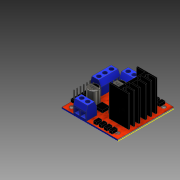
# Autodesk Inventor part: cau h l298
Saved by Autodesk Inventor 2016 (Build 200138000, 138)
## iProperties
Created: 2017-05-27
Part Number: cau h l298
Material: Generic
Document SubType Name: Modeling
Designer: USER
Density: 1 g/cm^3
Appearance: Default
Author: USER
Autodesk Inventor part; units mm, degrees
(part 1 of 2)
ref_plane "YZ Plane" through (0, 0, 0) normal (1, 0, 0) x (0, 1, 0)
sketch "Sketch1" plane through (0, 0, 0) normal (0, 0, 1) x (1, 0, 0)
  line L0 (-21.65, 21.65) -> (21.65, 21.65)
  line L1 (21.65, 21.65) -> (21.65, -21.65)
  line L2 (21.65, -21.65) -> (-21.65, -21.65)
  line L3 (-21.65, -21.65) -> (-21.65, 21.65)
  line L4 (0, 76.4696) -> (0, -38.0033) construction
  line L5 (-31.8613, 0) -> (39.6177, 0) construction
  circle A0 centre (-17.8322, 17.7673) radius 1.5
  circle A1 centre (-17.8322, -17.8659) radius 1.5
  circle A2 centre (17.7069, 17.7673) radius 1.5
  circle A3 centre (17.2358, -17.5058) radius 1.5
  line L6 (14.4064, 60.1163) -> (29.4064, 60.1163)
  line L7 (21.65, 11) -> (21.65, -11)
  line L8 (29.4064, 38.1163) -> (14.4064, 38.1163)
  line L9 (14.4064, 38.1163) -> (14.4064, 60.1163)
  line L10 (20.9064, 60.1163) -> (20.9064, 38.1163)
  line L11 (23.3464, 51.1163) -> (23.3464, 47.1163)
  arc A4 (23.6564, 58.1213) -> (23.6564, 57.1113) centre (23.6564, 57.6163) ccw
  arc A5 (23.6564, 41.1213) -> (23.6564, 40.1113) centre (23.6564, 40.6163) ccw
  line L12 (14.4064, 59.1163) -> (20.9064, 59.1163)
  line L13 (23.6564, 59.1163) -> (29.4064, 59.1163)
  line L14 (14.4064, 56.1163) -> (20.9064, 56.1163)
  line L15 (23.6564, 56.1163) -> (29.4064, 56.1163)
  line L16 (14.4064, 55.1163) -> (20.9064, 55.1163)
  line L17 (21.9064, 55.1163) -> (29.4064, 55.1163)
  line L18 (21.9064, 55.1163) -> (21.9064, 52.1163)
  line L19 (14.4064, 51.1163) -> (20.9064, 51.1163)
  line L20 (23.3464, 51.1163) -> (29.4064, 51.1163)
  line L21 (14.4064, 47.1163) -> (20.9064, 47.1163)
  line L22 (23.3464, 47.1163) -> (29.4064, 47.1163)
  line L23 (14.4064, 43.1163) -> (20.9064, 43.1163)
  line L24 (21.9064, 43.1163) -> (29.4064, 43.1163)
  line L25 (14.4064, 46.1163) -> (20.9064, 46.1163)
  line L26 (21.9064, 46.1163) -> (29.4064, 46.1163)
  line L27 (21.9064, 46.1163) -> (21.9064, 43.1163)
  line L28 (14.4064, 42.1163) -> (20.9064, 42.1163)
  line L29 (23.6564, 42.1163) -> (29.4064, 42.1163)
  line L30 (14.4064, 39.1163) -> (20.9064, 39.1163)
  line L31 (23.6564, 39.1163) -> (29.4064, 39.1163)
  line L32 (14.4064, 52.1163) -> (20.9064, 52.1163)
  line L33 (21.9064, 52.1163) -> (29.4064, 52.1163)
  line L34 (23.6564, 59.1163) -> (23.6564, 58.1213)
  line L35 (23.6564, 57.1113) -> (23.6564, 56.1163)
  line L36 (23.6564, 42.1163) -> (23.6564, 41.1213)
  line L37 (23.6564, 40.1113) -> (23.6564, 39.1163)
  point P0 (0, 0)
  point P1 (21.9064, 60.1163)
  point P2 (21.9064, 38.1163)
  dimension "d0" = 43.3
  dimension "d1" = 43.3
  dimension "d2" = 3
  dimension "d3" = 3
  dimension "d4" = 3
  dimension "d5" = 3
  dimension "d6" = 15
  dimension "d7" = 22
  dimension "d23" = 1.01
  dimension "d24" = 1.01
  constraints: 70 end point, 36 parallel, 14 perpendicular, 6 centre point, 4 point on circle, 2 horizontal, 2 midpoint, 2 point on line, 2 vertical, 1 collinear, 15 other
  measures "d0" distance of L1.end L2.end
  measures "d1" distance of L0.end L1.end
  measures "d2" diameter of A0
  measures "d3" diameter of A1
  measures "d4" diameter of A2
  measures "d5" diameter of A3
  measures "d6" distance of L8.start L8.end
  measures "d7" distance of L7.start L7.end
  measures "d23" diameter of A4
  measures "d24" diameter of A5
extrude "Extrusion1" [suppressed]
extrude "Extrusion2" add sketch "Sketch1" along normal blind 1 contours L0 L1 L2 L3
sketch "Sketch2" plane through (0, 0, 1) normal (0, 0, 1) x (1, 0, 0)
  line L0 (4.3418, 10.9877) -> (19.3418, 10.9877)
  line L1 (19.3418, -11.0123) -> (4.3418, -11.0123)
  line L2 (10.8418, 9.9877) -> (10.8418, -10.0123)
  line L3 (13.2818, 1.9877) -> (13.2818, -2.0123)
  arc A0 (13.5918, 8.9927) -> (13.5918, 7.9827) centre (13.5918, 8.4877) ccw
  arc A1 (13.5918, -8.0073) -> (13.5918, -9.0173) centre (13.5918, -8.5123) ccw
  line L4 (4.3418, 9.9877) -> (10.8418, 9.9877)
  line L5 (13.5918, 9.9877) -> (19.3418, 9.9877)
  line L6 (13.5918, 6.9877) -> (19.3418, 6.9877)
  line L7 (11.8418, 5.9877) -> (19.3418, 5.9877)
  line L8 (11.8418, 5.9877) -> (11.8418, 2.9877)
  line L9 (13.2818, 1.9877) -> (19.3418, 1.9877)
  line L10 (13.2818, -2.0123) -> (19.3418, -2.0123)
  line L11 (11.8412, -6.1108) -> (19.3409, -6.1108)
  line L12 (11.8412, -3.1108) -> (19.3418, -3.1108)
  line L13 (11.8412, -3.1108) -> (11.8412, -6.1108)
  line L14 (13.5918, -7.0123) -> (19.3418, -7.0123)
  line L15 (4.3418, -10.0123) -> (10.8418, -10.0123)
  line L16 (13.5918, -10.0123) -> (19.3418, -10.0123)
  line L17 (11.8418, 2.9877) -> (19.3418, 2.9877)
  line L18 (13.5918, 9.9877) -> (13.5918, 8.9927)
  line L19 (13.5918, 7.9827) -> (13.5918, 6.9877)
  line L20 (13.5918, -7.0123) -> (13.5918, -8.0073)
  line L21 (13.5918, -9.0173) -> (13.5918, -10.0123)
  line L22 (20.4576, -0.0123) -> (1.0901, -0.0123) construction
  line L23 (21.65, -21.65) -> (21.65, 21.65) projected
  circle A2 centre (17.2358, -17.5058) radius 1.5 projected
  circle A3 centre (17.7069, 17.7673) radius 1.5 projected
  circle A4 centre (-17.8322, -17.8659) radius 1.5 projected
  circle A5 centre (-17.8322, 17.7673) radius 1.5 projected
  line L24 (21.65, 21.65) -> (-21.65, 21.65)
  line L25 (32.7891, 0) -> (-24.0691, 0) construction
  line L26 (0, 31.3207) -> (0, -29.8157) construction
  line L27 (19.3418, 0) -> (19.3418, -0.0123)
  line L28 (19.3418, 10.9877) -> (19.3418, 9.9877)
  line L29 (19.3418, 6.9877) -> (19.3418, 5.9877)
  line L30 (19.3418, 2.9877) -> (19.3418, 1.9877)
  line L31 (19.3418, -2.0123) -> (19.3418, -3.1108)
  line L32 (19.3418, -6.1108) -> (19.3418, -7.0123)
  line L33 (19.3418, -10.0123) -> (19.3418, -11.0969)
  line L34 (4.3418, 9.9877) -> (4.3418, 10.9877)
  line L35 (4.3418, -11.0123) -> (4.3418, -10.0123)
  line L36 (4.3418, -0.0123) -> (4.3418, 0)
  line L37 (19.3418, 10.9877) -> (19.3418, 9.9877)
  line L38 (13.5918, 9.9877) -> (13.5918, 8.9927)
  line L39 (13.5918, 6.9877) -> (19.3418, 6.9877)
  line L40 (19.3418, 5.9877) -> (11.8418, 5.9877)
  line L41 (11.8418, 2.9877) -> (19.3418, 2.9877)
  line L42 (19.3418, 1.9877) -> (13.2818, 1.9877)
  line L43 (4.3418, 10.9877) -> (19.3418, 10.9877)
  line L44 (19.3418, 10.9877) -> (19.3418, 9.9877)
  line L45 (19.3418, 9.9877) -> (13.5918, 9.9877)
  line L46 (13.5918, 9.9877) -> (13.5918, 8.9927)
  line L47 (13.5918, 7.9827) -> (13.5918, 6.9877)
  line L48 (13.5918, 6.9877) -> (19.3418, 6.9877)
  line L49 (19.3418, 6.9877) -> (19.3418, 5.9877)
  line L50 (19.3418, 5.9877) -> (11.8418, 5.9877)
  line L51 (11.8418, 5.9877) -> (11.8418, 2.9877)
  line L52 (11.8418, 2.9877) -> (19.3418, 2.9877)
  line L53 (19.3418, 2.9877) -> (19.3418, 1.9877)
  line L54 (19.3418, 1.9877) -> (13.2818, 1.9877)
  line L55 (13.2818, 1.9877) -> (13.2818, -2.0123)
  line L56 (13.2818, -2.0123) -> (19.3418, -2.0123)
  line L57 (19.3418, -3.1108) -> (19.3418, -2.0123)
  line L58 (19.3418, -3.1108) -> (11.8412, -3.1108)
  line L59 (11.8412, -3.1108) -> (11.8412, -6.1108)
  line L60 (11.8412, -6.1108) -> (19.3418, -6.1108)
  line L61 (19.3418, -6.1108) -> (19.3418, -7.0123)
  line L62 (19.3418, -7.0123) -> (13.5918, -7.0123)
  line L63 (13.5918, -7.0123) -> (13.5918, -8.0073)
  line L64 (13.5918, -9.0173) -> (13.5918, -10.0123)
  line L65 (13.5918, -10.0123) -> (19.3418, -10.0123)
  line L66 (19.3418, -10.0123) -> (19.3418, -11.0123)
  line L67 (19.3418, -11.0123) -> (4.3418, -11.0123)
  line L68 (4.3418, -11.0123) -> (4.3418, -10.0123)
  line L69 (4.3418, -10.0123) -> (10.8418, -10.0123)
  line L70 (10.8418, -10.0123) -> (10.8418, 9.9877)
  line L71 (10.8418, 9.9877) -> (4.3418, 9.9877)
  line L72 (4.3418, 9.9877) -> (4.3418, 10.9877)
  line L73 (4.3418, 10.9877) -> (19.3418, 10.9877)
  arc A6 (13.5918, 8.9927) -> (13.5918, 7.9827) centre (13.5918, 8.4877) ccw
  arc A7 (13.5918, -8.0073) -> (13.5918, -9.0173) centre (13.5918, -8.5123) ccw
  point P0 (0, 0)
  point P1 (11.8418, 10.9877)
  point P2 (11.8418, -11.0123)
  dimension "d29" = 15
  dimension "d30" = 1.01
  dimension "d31" = 1.01
  constraints: 146 end point, 26 collinear, 16 perpendicular, 15 parallel, 8 centre point, 8 point on circle, 6 point on line, 5 vertical, 3 horizontal, 2 concentric, 2 midpoint
  measures "d29" distance of L1.start L1.end
  measures "d30" diameter of A0
  measures "d31" diameter of A1
extrude "Extrusion3" add sketch "Sketch2" along normal blind 24 contours L0 L28 L5 L18 A0 L19 L6 L29 L7 L8 L17 L30 L9 L3 L10 L31 L12 L13 L11 L32 L14 L20 A1 L21 L16 L33 L1 L35 L15 L2 L4 L34
sketch "Sketch3" plane through (10.8418, -10.0123, 1) normal (-1, 0, 0) x (0, 0, 1)
  line L0 (24, 20) -> (24, 0) projected
  line L1 (0, 0) -> (24, 0) projected
  line L2 (0, 20) -> (24, 20) projected
  line L3 (0, 31.6623) -> (0, -11.6377) projected
  line L4 (24, 10) -> (0, 10) construction
  line L5 (0, 0) -> (0, 20) construction
  line L6 (21.15, 16.985) -> (21.15, 3.015)
  line L7 (21.15, 3.015) -> (19.14, 3.015) construction
  line L8 (19.14, 3.015) -> (19.14, 1.005) construction
  line L9 (21.15, 16.985) -> (19.1401, 16.985) construction
  line L10 (19.1401, 16.985) -> (19.1401, 18.995) construction
  line L11 (21.15, 3.015) -> (19.14, 1.005)
  line L12 (21.15, 16.985) -> (19.1401, 18.995)
  line L13 (19.14, 1.005) -> (4.15, 1.005)
  line L14 (4.15, 1.005) -> (4.15, 18.995)
  line L15 (0, 0) -> (24, 0) projected
  line L16 (4.15, 18.995) -> (19.1401, 18.995)
  line L17 (0, 0.995) -> (24, 0.995) projected
  line L18 (15.15, 18.995) -> (15.15, 1.005)
  point P0 (-1, 10.0123)
  dimension "d34" = 13.97
  dimension "d35" = 2.01
  dimension "d36" = 2.01
  dimension "d37" = 2.0099
  dimension "d38" = 2.01
  dimension "d39" = 2.85
  dimension "d40" = 14.99
  dimension "d41" = 14.99
  dimension "d42" = 11
  constraints: 24 end point, 3 perpendicular, 2 midpoint, 2 point on line, 2 vertical, 1 horizontal, 1 symmetric about line
  measures "d34" distance of L6.start L6.end
  measures "d35" distance of L6.end L7.end
  measures "d36" distance of L7.end L8.end
  measures "d37" distance of L6.start L9.end
  measures "d38" distance of L9.end L10.end
  measures "d39" distance between parallel lines of L6 L0
  measures "d40" distance of L8.end L13.end
  measures "d41" distance of L8.end L13.end
  measures "d42" distance between parallel lines of L14 L18
extrude "Extrusion4" add sketch "Sketch3" along normal blind 2 contours L6 L11 L13 L18 L16 L12
extrude "Extrusion5" add sketch "Sketch3" along normal blind 5 contours L18 L13 L14 L16
sketch "Sketch4" plane through (5.8418, -10.0123, 1) normal (-1, 0, 0) x (0, 0, 1)
  line L0 (11.7643, 16.7385) -> (11.7643, 8.5437) construction
  line L1 (11.7643, 8.5437) -> (6.177, 8.5437) construction
  line L2 (6.177, 8.5437) -> (6.177, 16.7385) construction
  line L3 (6.177, 16.7385) -> (11.7643, 16.7385) construction
  point P0 (-1, 10.0123)
  constraints: 2 other
sketch "Sketch5" plane through (8.8418, -10.0123, 1) normal (-1, 0, 0) x (0, 0, 1)
  line L0 (24, 10) -> (0, 10) construction
  circle A0 centre (18.3207, 10) radius 1.5
  point P0 (-1, 10.0123)
  dimension "d47" = 3
  constraints: 1 centre point, 1 point on line
  measures "d47" diameter of A0
extrude "Extrusion6" cut sketch "Sketch5" against normal through all
sketch "Sketch6" plane through (0, 0, 1) normal (0, 0, 1) x (1, 0, 0)
  line L0 (16.09, -16.41) -> (13.59, -16.41)
  line L1 (13.59, -16.41) -> (13.59, -20.41)
  line L2 (13.59, -20.41) -> (16.09, -20.41)
  line L3 (16.09, -20.41) -> (16.09, -16.41)
  line L4 (21.65, -21.65) -> (21.65, 21.65) projected
  line L5 (-21.65, -21.65) -> (21.65, -21.65) projected
  line L6 (12.09, -16.41) -> (9.59, -16.41)
  line L7 (9.59, -16.41) -> (9.59, -20.41)
  line L8 (9.59, -20.41) -> (12.09, -20.41)
  line L9 (12.09, -20.41) -> (12.09, -16.41)
  line L10 (8.09, -16.41) -> (5.59, -16.41)
  line L11 (5.59, -16.41) -> (5.59, -20.41)
  line L12 (5.59, -20.41) -> (8.09, -20.41)
  line L13 (8.09, -20.41) -> (8.09, -16.41)
  line L14 (4.09, -16.41) -> (1.59, -16.41)
  line L15 (1.59, -16.41) -> (1.59, -20.41)
  line L16 (1.59, -20.41) -> (4.09, -20.41)
  line L17 (4.09, -20.41) -> (4.09, -16.41)
  line L18 (4.3418, -11.0123) -> (4.3418, -10.0123) construction
  line L19 (4.3418, -10.0123) -> (10.8418, -10.0123) construction
  line L20 (10.8418, -10.0123) -> (10.8418, 9.9877) construction
  line L21 (10.8418, 9.9877) -> (4.3418, 9.9877) construction
  line L22 (4.3418, 9.9877) -> (4.3418, 10.9877) construction
  line L23 (4.3418, 10.9877) -> (19.3418, 10.9877) construction
  line L24 (19.3418, 10.9877) -> (19.3418, 9.9877) construction
  line L25 (19.3418, 9.9877) -> (13.5918, 9.9877) construction
  line L26 (13.5918, 9.9877) -> (13.5918, 8.9927) construction
  arc A0 (13.5918, 8.9927) -> (13.5918, 7.9827) centre (13.5918, 8.4877) ccw construction
  line L27 (13.5918, 7.9827) -> (13.5918, 6.9877) construction
  line L28 (13.5918, 6.9877) -> (19.3418, 6.9877) construction
  line L29 (19.3418, 6.9877) -> (19.3418, 5.9877) construction
  line L30 (19.3418, 5.9877) -> (11.8418, 5.9877) construction
  line L31 (11.8418, 5.9877) -> (11.8418, 2.9877) construction
  line L32 (11.8418, 2.9877) -> (19.3418, 2.9877) construction
  line L33 (19.3418, 2.9877) -> (19.3418, 1.9877) construction
  line L34 (19.3418, 1.9877) -> (13.2818, 1.9877) construction
  line L35 (13.2818, 1.9877) -> (13.2818, -2.0123) construction
  line L36 (13.2818, -2.0123) -> (19.3418, -2.0123) construction
  line L37 (19.3418, -2.0123) -> (19.3418, -3.1108) construction
  line L38 (19.3418, -3.1108) -> (11.8412, -3.1108) construction
  line L39 (11.8412, -3.1108) -> (11.8412, -6.1108) construction
  line L40 (11.8412, -6.1108) -> (19.3418, -6.1108) construction
  line L41 (19.3418, -6.1108) -> (19.3418, -7.0123) construction
  line L42 (19.3418, -7.0123) -> (13.5918, -7.0123) construction
  line L43 (13.5918, -7.0123) -> (13.5918, -8.0073) construction
  arc A1 (13.5918, -8.0073) -> (13.5918, -9.0173) centre (13.5918, -8.5123) ccw construction
  line L44 (13.5918, -9.0173) -> (13.5918, -10.0123) construction
  line L45 (13.5918, -10.0123) -> (19.3418, -10.0123) construction
  line L46 (19.3418, -10.0123) -> (19.3418, -11.0123) construction
  line L47 (19.3418, -11.0123) -> (4.3418, -11.0123) construction
  circle A2 centre (17.2358, -17.5058) radius 1.5 construction
  circle A3 centre (17.7069, 17.7673) radius 1.5 construction
  circle A4 centre (-17.8322, -17.8659) radius 1.5 construction
  circle A5 centre (-17.8322, 17.7673) radius 1.5 construction
  line L48 (21.65, 21.65) -> (-21.65, 21.65) construction
  line L49 (-21.65, 21.65) -> (-21.65, -21.65) construction
  line L50 (-21.65, -21.65) -> (21.65, -21.65) construction
  line L51 (21.65, -21.65) -> (21.65, 21.65) construction
  line L52 (19.7772, 0) -> (14.3327, 0) construction
  line L53 (16.09, 16.41) -> (13.59, 16.41)
  line L54 (13.59, 16.41) -> (13.59, 20.41)
  line L55 (13.59, 20.41) -> (16.09, 20.41)
  line L56 (16.09, 20.41) -> (16.09, 16.41)
  line L57 (12.09, 16.41) -> (9.59, 16.41)
  line L58 (9.59, 16.41) -> (9.59, 20.41)
  line L59 (9.59, 20.41) -> (12.09, 20.41)
  line L60 (12.09, 20.41) -> (12.09, 16.41)
  line L61 (8.09, 16.41) -> (5.59, 16.41)
  line L62 (5.59, 16.41) -> (5.59, 20.41)
  line L63 (5.59, 20.41) -> (8.09, 20.41)
  line L64 (8.09, 20.41) -> (8.09, 16.41)
  line L65 (4.09, 16.41) -> (1.59, 16.41)
  line L66 (1.59, 16.41) -> (1.59, 20.41)
  line L67 (1.59, 20.41) -> (4.09, 20.41)
  line L68 (4.09, 20.41) -> (4.09, 16.41)
  line L69 (-2.65, -13.65) -> (-12.65, -13.65)
  line L70 (-12.65, -13.65) -> (-12.65, -21.65)
  line L71 (-12.65, -21.65) -> (-2.65, -21.65)
  line L72 (-2.65, -21.65) -> (-2.65, -13.65)
  line L73 (-13.65, 15.65) -> (-21.65, 15.65)
  line L74 (-21.65, 15.65) -> (-21.65, 0.65)
  line L75 (-21.65, 0.65) -> (-13.65, 0.65)
  line L76 (-13.65, 0.65) -> (-13.65, 15.65)
  line L77 (-21.65, 21.65) -> (-21.65, -21.65) projected
  line L78 (-21.65, 0.26) -> (-21.65, -14.74)
  line L79 (-21.65, -14.74) -> (-16.65, -14.74)
  line L80 (-16.65, -14.74) -> (-16.65, -12.24)
  line L81 (-16.65, -12.24) -> (-19.15, -12.24)
  line L82 (-19.15, -12.24) -> (-19.15, -2.24)
  line L83 (-19.15, -2.24) -> (-16.65, -2.24)
  line L84 (-16.65, -2.24) -> (-16.65, 0.26)
  line L85 (-16.65, 0.26) -> (-21.65, 0.26)
  line L86 (-16.65, 0.26) -> (-21.65, 0.26)
  line L87 (-21.65, 0.26) -> (-21.65, -14.74)
  line L88 (-21.65, -14.74) -> (-16.65, -14.74)
  line L89 (-16.65, -14.74) -> (-16.65, 0.26)
  line L90 (-16.65, -2.24) -> (-19.15, -2.24)
  line L91 (-19.15, -2.24) -> (-19.15, -12.24)
  line L92 (-19.15, -12.24) -> (-16.65, -12.24)
  line L93 (-10.15, 12) -> (-12.65, 12)
  line L94 (-12.65, 12) -> (-12.65, 7)
  line L95 (-12.65, 7) -> (-10.15, 7)
  line L96 (-10.15, 7) -> (-10.15, 12)
  line L97 (-11.15, 11) -> (-11.65, 11)
  line L98 (-11.65, 11) -> (-11.65, 10.5)
  line L99 (-11.65, 10.5) -> (-11.15, 10.5)
  line L100 (-11.15, 10.5) -> (-11.15, 11)
  line L101 (-11.15, 8.5) -> (-11.65, 8.5)
  line L102 (-11.65, 8.5) -> (-11.65, 8)
  line L103 (-11.65, 8) -> (-11.15, 8)
  line L104 (-11.15, 8) -> (-11.15, 8.5)
  circle A6 centre (-13, -6) radius 4
  circle A7 centre (-5, 6.4877) radius 4
  line L105 (1.0618, -7.2823) -> (0.5618, -7.2823)
  line L106 (0.5618, -7.2823) -> (0.5618, -7.7823)
  line L107 (0.5618, -7.7823) -> (1.0618, -7.7823)
  line L108 (1.0618, -7.7823) -> (1.0618, -7.2823)
  line L109 (5.8418, -9.0073) -> (5.8418, 8.9827) projected
  line L110 (1.0618, -5.7823) -> (1.0618, -5.2823)
  line L111 (1.0618, -5.2823) -> (0.5618, -5.2823)
  line L112 (0.5618, -5.2823) -> (0.5618, -5.7823)
  line L113 (0.5618, -5.7823) -> (1.0618, -5.7823)
  line L114 (1.0618, -3.7823) -> (1.0618, -3.2823)
  line L115 (1.0618, -3.2823) -> (0.5618, -3.2823)
  line L116 (0.5618, -3.2823) -> (0.5618, -3.7823)
  line L117 (0.5618, -3.7823) -> (1.0618, -3.7823)
  line L118 (1.0618, -1.7823) -> (1.0618, -1.2823)
  line L119 (1.0618, -1.2823) -> (0.5618, -1.2823)
  line L120 (0.5618, -1.2823) -> (0.5618, -1.7823)
  line L121 (0.5618, -1.7823) -> (1.0618, -1.7823)
  line L122 (1.0618, 0.2177) -> (1.0618, 0.7177)
  line L123 (1.0618, 0.7177) -> (0.5618, 0.7177)
  line L124 (0.5618, 0.7177) -> (0.5618, 0.2177)
  line L125 (0.5618, 0.2177) -> (1.0618, 0.2177)
  line L126 (1.0618, 2.2177) -> (1.0618, 2.7177)
  line L127 (1.0618, 2.7177) -> (0.5618, 2.7177)
  line L128 (0.5618, 2.7177) -> (0.5618, 2.2177)
  line L129 (0.5618, 2.2177) -> (1.0618, 2.2177)
  line L130 (1.0618, 4.2177) -> (1.0618, 4.7177)
  line L131 (1.0618, 4.7177) -> (0.5618, 4.7177)
  line L132 (0.5618, 4.7177) -> (0.5618, 4.2177)
  line L133 (0.5618, 4.2177) -> (1.0618, 4.2177)
  line L134 (1.0618, 6.2177) -> (1.0618, 6.7177)
  line L135 (1.0618, 6.7177) -> (0.5618, 6.7177)
  line L136 (0.5618, 6.7177) -> (0.5618, 6.2177)
  line L137 (0.5618, 6.2177) -> (1.0618, 6.2177)
  line L138 (7.5918, -6.2823) -> (7.0918, -6.2823)
  line L139 (7.0918, -6.2823) -> (7.0918, -6.7823)
  line L140 (7.0918, -6.7823) -> (7.5918, -6.7823)
  line L141 (7.5918, -6.7823) -> (7.5918, -6.2823)
  line L142 (7.0918, -4.2823) -> (7.0918, -4.7823)
  line L143 (7.0918, -4.7823) -> (7.5918, -4.7823)
  line L144 (7.5918, -4.7823) -> (7.5918, -4.2823)
  line L145 (7.5918, -4.2823) -> (7.0918, -4.2823)
  line L146 (7.0918, -2.2823) -> (7.0918, -2.7823)
  line L147 (7.0918, -2.7823) -> (7.5918, -2.7823)
  line L148 (7.5918, -2.7823) -> (7.5918, -2.2823)
  line L149 (7.5918, -2.2823) -> (7.0918, -2.2823)
  line L150 (7.0918, -0.2823) -> (7.0918, -0.7823)
  line L151 (7.0918, -0.7823) -> (7.5918, -0.7823)
  line L152 (7.5918, -0.7823) -> (7.5918, -0.2823)
  line L153 (7.5918, -0.2823) -> (7.0918, -0.2823)
  line L154 (7.0918, 1.7177) -> (7.0918, 1.2177)
  line L155 (7.0918, 1.2177) -> (7.5918, 1.2177)
  line L156 (7.5918, 1.2177) -> (7.5918, 1.7177)
  line L157 (7.5918, 1.7177) -> (7.0918, 1.7177)
  line L158 (7.0918, 3.7177) -> (7.0918, 3.2177)
  line L159 (7.0918, 3.2177) -> (7.5918, 3.2177)
  line L160 (7.5918, 3.2177) -> (7.5918, 3.7177)
  line L161 (7.5918, 3.7177) -> (7.0918, 3.7177)
  line L162 (7.0918, 5.7177) -> (7.0918, 5.2177)
  line L163 (7.0918, 5.2177) -> (7.5918, 5.2177)
  line L164 (7.5918, 5.2177) -> (7.5918, 5.7177)
  line L165 (7.5918, 5.7177) -> (7.0918, 5.7177)
  line L166 (7.0918, 7.7177) -> (7.0918, 7.2177)
  line L167 (7.0918, 7.2177) -> (7.5918, 7.2177)
  line L168 (7.5918, 7.2177) -> (7.5918, 7.7177)
  line L169 (7.5918, 7.7177) -> (7.0918, 7.7177)
  line L170 (-1.8244, -4.6108) -> (-7.65, -4.6108)
  line L171 (-7.65, -4.6108) -> (-7.65, -10)
  line L172 (-7.65, -10) -> (-1.8244, -10)
  line L173 (-1.8244, -10) -> (-1.8244, -4.6108)
  point P0 (0, 0)
  point P1 (-21.65, 8.15)
  dimension "d50" = 2.5
  dimension "d51" = 4
  dimension "d52" = 5.56
  dimension "d53" = 1.24
  dimension "d56" = 4
  dimension "d63" = 10
  dimension "d64" = 8
  dimension "d65" = 9
  dimension "d85" = 8
  dimension "d86" = 15
  dimension "d87" = 6
  dimension "d109" = 15
  dimension "d110" = 5
  dimension "d111" = 2.5
  dimension "d112" = 2.5
  dimension "d113" = 10
  dimension "d114" = 2.5
  dimension "d115" = 2.5
  dimension "d116" = 6.91
  dimension "d154" = 2.5
  dimension "d155" = 5
  dimension "d156" = 1
  dimension "d157" = 0.5
  dimension "d158" = 0.5
  dimension "d159" = 1
  dimension "d160" = 1
  dimension "d165" = 0.5
  dimension "d166" = 0.5
  dimension "d167" = 1
  dimension "d168" = 1
  dimension "d173" = 8
  dimension "d178" = 8
  dimension "d182" = 0.5
  dimension "d183" = 0.5
  dimension "d184" = 2.23
  dimension "d185" = 4.78
  dimension "d188" = 2
  dimension "d193" = 0.5
  dimension "d194" = 0.5
  dimension "d195" = 0.5
  dimension "d198" = 2
  constraints: 272 end point, 21 equal length, 16 symmetric about line, 14 perpendicular, 12 horizontal, 6 point on line, 3 collinear, 2 centre point, 2 vertical, 1 midpoint, 133 other
  measures "d50" distance of L2.end L1.end
  measures "d51" distance of L1.end L0.end
  measures "d52" distance between parallel lines of L4 L3
  measures "d53" distance between parallel lines of L5 L2
  measures "d56" distance of L0.start L6.start
  measures "d63" distance of L71.end L70.end
  measures "d64" distance of L70.end L69.end
  measures "d65" distance between parallel lines of L49 L70
  measures "d85" distance of L75.end L74.end
  measures "d86" distance of L74.end L73.end
  measures "d87" distance between parallel lines of L48 L73
  measures "d109" distance of L78.start L78.end
  measures "d110" distance of L78.end L79.end
  measures "d111" distance of L79.end L80.end
  measures "d112" distance of L80.end L81.end
  measures "d113" distance of L81.end L82.end
  measures "d114" distance of L82.end L83.end
  measures "d115" distance of L83.end L84.end
  measures "d116" distance between parallel lines of L5 L79
  measures "d154" distance of L95.end L94.end
  measures "d155" distance of L94.end L93.end
  measures "d156" distance between parallel lines of L76 L94
  measures "d157" distance of L99.end L98.end
  measures "d158" distance of L98.end L97.end
  measures "d159" distance between parallel lines of L96 L100
  measures "d160" distance between parallel lines of L93 L97
  measures "d165" distance of L103.end L102.end
  measures "d166" distance of L102.end L101.end
  measures "d167" distance between parallel lines of L95 L103
  measures "d168" distance between parallel lines of L94 L102
  measures "d173" diameter of A6
  measures "d178" diameter of A7
  measures "d182" distance of L107.end L106.end
  measures "d183" distance of L106.end L105.end
  measures "d184" distance between parallel lines of L107 L19
  measures "d185" distance between parallel lines of L108 L109
  measures "d188" distance of L105.start L110.end
  measures "d193" distance of L140.end L139.end
  measures "d194" distance of L139.end L138.end
  measures "d195" distance from line of L105.start L140
  measures "d198" distance of L138.end L142.start
extrude "Extrusion7" add sketch "Sketch6" along normal blind 2 contours L3 L2 L1 L0 | L9 L8 L7 L6 | L13 L12 L11 L10 | L17 L16 L15 L14 | L53 L54 L55 L56 | L57 L58 L59 L60 | L61 L62 L63 L64 | L65 L66 L67 L68
extrude "Extrusion8" add sketch "Sketch6" along normal blind 6 contours L70 L69 L72 L5
sketch "Sketch7" plane through (-21.65, -21.65, 0) normal (0, -1, 0) x (1, 0, 0)
  line L0 (9.7004, 6) -> (13.7004, 6)
  line L1 (13.7004, 6) -> (13.7004, 2)
  line L2 (13.7004, 2) -> (9.7004, 2)
  line L3 (9.7004, 2) -> (9.7004, 6)
  line L4 (14.2828, 6) -> (18.2828, 6)
  line L5 (18.2828, 6) -> (18.2828, 2)
  line L6 (18.2828, 2) -> (14.2828, 2)
  line L7 (14.2828, 2) -> (14.2828, 6)
  point P0 (21.65, 0)
  dimension "d68" = 4
  dimension "d69" = 4
  dimension "d70" = 4
  dimension "d71" = 4
  constraints: 16 end point, 4 parallel, 2 horizontal, 2 perpendicular
  measures "d68" distance of L1.end L2.end
  measures "d69" distance of L0.end L1.end
  measures "d70" distance of L5.end L6.end
  measures "d71" distance of L4.end L5.end
extrude "Extrusion9" cut sketch "Sketch7" against normal blind 4
ref_plane "Work Plane1" through (0, 0, 11) normal (0, 0, 1) x (1, 0, 0)
sketch "Sketch8" plane through (0, 0, 11) normal (0, 0, 1) x (1, 0, 0)
  line L0 (-12.65, -15.4024) -> (-2.65, -15.4024)
  line L1 (-2.65, -15.4024) -> (-2.65, -20.7624)
  line L2 (-2.65, -20.7624) -> (-12.65, -20.7624)
  line L3 (-12.65, -20.7624) -> (-12.65, -15.4024)
  point P0 (0, 0)
  dimension "d75" = 10
  dimension "d76" = 5.36
  constraints: 8 end point, 2 parallel, 1 horizontal, 1 perpendicular
  measures "d75" distance of L1.end L2.end
  measures "d76" distance of L0.end L1.end
sketch "Sketch9" plane through (0, 0, 7) normal (0, 0, 1) x (1, 0, 0)
  line L0 (-12.65, -21.65) -> (-2.65, -21.65) projected
  line L1 (-12.65, -13.65) -> (-12.65, -21.65) projected
  line L2 (-2.65, -13.65) -> (-12.65, -13.65) projected
  line L3 (-2.65, -21.65) -> (-2.65, -13.65) projected
  point P0 (0, 0)
loft "Loft1" add profiles "Sketch8" section 1 edges at (-7.65, -13.65, 7) (-12.65, -17.65, 7) (-7.65, -21.65, 7) (-2.65, -17.65, 7)
sketch "Sketch10" plane through (-12.65, -15.4024, 11) normal (0, 0, 1) x (1, 0, 0)
  circle A0 centre (7.2601, -2.5465) radius 1.5
  circle A1 centre (2.6528, -2.5465) radius 1.5
  point P0 (12.65, 15.4024)
  dimension "d81" = 3
  dimension "d82" = 3
  constraints: 2 centre point
  measures "d81" diameter of A0
  measures "d82" diameter of A1
extrude "Extrusion10" cut sketch "Sketch10" against normal blind 2
mirror "Mirror1" about plane through (0, 0, 0) normal (0, 1, 0) of "Extrusion10", "Loft1", "Extrusion8", "Extrusion9"
extrude "Extrusion11" add sketch "Sketch6" along normal blind 6 contours L76 L75 L74 L73
ref_plane "Work Plane2" through (0, 0, 11) normal (0, 0, 1) x (1, 0, 0)
sketch "Sketch12" plane through (-21.65, -21.65, 0) normal (-1, 0, 0) x (0, 0, 1)
  line L0 (6, 36.5283) -> (2, 36.5283)
  line L1 (2, 36.5283) -> (2, 32.5283)
  line L2 (2, 32.5283) -> (6, 32.5283)
  line L3 (6, 32.5283) -> (6, 36.5283)
  line L4 (6, 31.7395) -> (2, 31.7395)
  line L5 (2, 31.7395) -> (2, 27.7395)
  line L6 (2, 27.7395) -> (6, 27.7395)
  line L7 (6, 27.7395) -> (6, 31.7395)
  line L8 (6, 26.993) -> (2, 26.993)
  line L9 (2, 26.993) -> (2, 22.993)
  line L10 (2, 22.993) -> (6, 22.993)
  line L11 (6, 22.993) -> (6, 26.993)
  point P0 (0, 21.65)
  dimension "d96" = 4
  dimension "d97" = 4
  dimension "d98" = 4
  dimension "d99" = 4
  dimension "d100" = 4
  dimension "d101" = 4
  constraints: 24 end point, 6 parallel, 3 horizontal, 3 perpendicular
  measures "d96" distance of L2.end L1.end
  measures "d97" distance of L1.end L0.end
  measures "d98" distance of L6.end L5.end
  measures "d99" distance of L5.end L4.end
  measures "d100" distance of L10.end L10.start
  measures "d101" distance of L10.start L9.start
extrude "Extrusion12" cut sketch "Sketch12" against normal blind 4
extrude "Extrusion14" add sketch "Sketch6" along normal blind 2 contours L85 L84 L83 L82 L81 L80 L79 L77
sketch "Sketch14" plane through (0, 0, 3) normal (0, 0, 1) x (1, 0, 0)
  line L0 (-17.65, -13.24) -> (-18.15, -13.24)
  line L1 (-18.15, -13.24) -> (-18.15, -13.74)
  line L2 (-18.15, -13.74) -> (-17.65, -13.74)
  line L3 (-17.65, -13.74) -> (-17.65, -13.24)
  line L4 (-16.65, -14.74) -> (-16.65, -12.24) projected
  line L5 (-16.65, -12.24) -> (-19.15, -12.24) projected
  line L6 (-20.15, -13.24) -> (-20.65, -13.24)
  line L7 (-20.65, -13.24) -> (-20.65, -13.74)
  line L8 (-20.65, -13.74) -> (-20.15, -13.74)
  line L9 (-20.15, -13.74) -> (-20.15, -13.24)
  line L10 (-21.65, -14.74) -> (-16.65, -14.74) projected
  line L11 (-21.65, 0.26) -> (-21.65, -14.74) projected
  line L12 (-20.15, -11.24) -> (-20.15, -10.74)
  line L13 (-20.65, -10.74) -> (-20.65, -11.24)
  line L14 (-20.65, -11.24) -> (-20.15, -11.24)
  line L15 (-20.15, -10.74) -> (-20.65, -10.74)
  line L16 (-20.15, -8.74) -> (-20.15, -8.24)
  line L17 (-20.65, -8.24) -> (-20.65, -8.74)
  line L18 (-20.65, -8.74) -> (-20.15, -8.74)
  line L19 (-20.15, -8.24) -> (-20.65, -8.24)
  line L20 (-20.15, -6.24) -> (-20.15, -5.74)
  line L21 (-20.65, -5.74) -> (-20.65, -6.24)
  line L22 (-20.65, -6.24) -> (-20.15, -6.24)
  line L23 (-20.15, -5.74) -> (-20.65, -5.74)
  line L24 (-20.15, -3.74) -> (-20.15, -3.24)
  line L25 (-20.65, -3.24) -> (-20.65, -3.74)
  line L26 (-20.65, -3.74) -> (-20.15, -3.74)
  line L27 (-20.15, -3.24) -> (-20.65, -3.24)
  line L28 (-20.15, -1.24) -> (-20.15, -0.74)
  line L29 (-20.65, -0.74) -> (-20.65, -1.24)
  line L30 (-20.65, -1.24) -> (-20.15, -1.24)
  line L31 (-20.15, -0.74) -> (-20.65, -0.74)
  line L32 (-17.65, -0.74) -> (-18.15, -0.74)
  line L33 (-18.15, -0.74) -> (-18.15, -1.24)
  line L34 (-18.15, -1.24) -> (-17.65, -1.24)
  line L35 (-17.65, -1.24) -> (-17.65, -0.74)
  line L36 (-19.15, -2.24) -> (-16.65, -2.24) projected
  line L37 (-16.65, -2.24) -> (-16.65, 0.26) projected
  point P0 (0, 0)
  dimension "d119" = 0.5
  dimension "d120" = 0.5
  dimension "d121" = 1
  dimension "d122" = 1
  dimension "d123" = 0.5
  dimension "d124" = 0.5
  dimension "d125" = 1
  dimension "d126" = 1
  dimension "d129" = 2.5
  dimension "d138" = 0.5
  dimension "d139" = 0.5
  dimension "d140" = 1
  dimension "d141" = 1
  constraints: 64 end point, 6 parallel, 3 horizontal, 3 perpendicular, 1 collinear, 1 vertical, 39 other
  measures "d119" distance of L2.end L1.end
  measures "d120" distance of L1.end L0.end
  measures "d121" distance between parallel lines of L3 L4
  measures "d122" distance between parallel lines of L5 L0
  measures "d123" distance of L8.end L7.end
  measures "d124" distance of L7.end L6.end
  measures "d125" distance between parallel lines of L10 L8
  measures "d126" distance between parallel lines of L11 L7
  measures "d129" distance of L6.start L12.end
  measures "d138" distance of L35.start L33.end
  measures "d139" distance of L33.end L33.start
  measures "d140" distance between parallel lines of L36 L34
  measures "d141" distance between parallel lines of L37 L35
sketch "Sketch15" plane through (0, 0, 7) normal (0, 0, 1) x (1, 0, 0)
  point P0 (0, 0)
sketch "Sketch16" plane through (0, 0, 11) normal (0, 0, 1) x (1, 0, 0)
  line L0 (-15.4501, 15.65) -> (-20.8101, 15.65)
  line L1 (-20.8101, 15.65) -> (-20.8101, 0.65)
  line L2 (-20.8101, 0.65) -> (-15.4501, 0.65)
  line L3 (-15.4501, 0.65) -> (-15.4501, 15.65)
  point P0 (0, 0)
  dimension "d142" = 5.36
  constraints: 8 end point, 2 parallel, 1 horizontal, 1 perpendicular
  measures "d142" distance of L2.end L1.end
loft "Loft3" add profiles "Sketch16" section 1 edges at (-17.65, 15.65, 7) (-21.65, 8.15, 7) (-17.65, 0.65, 7) (-13.65, 8.15, 7)
sketch "Sketch17" plane through (0, 0, 11) normal (0, 0, 1) x (1, 0, 0)
  circle A0 centre (-18, 13) radius 1.5
  circle A1 centre (-18, 8) radius 1.5
  circle A2 centre (-18, 3.3241) radius 1.5
  point P0 (0, 0)
  dimension "d147" = 3
  dimension "d148" = 3
  dimension "d149" = 3
  constraints: 3 centre point
  measures "d147" diameter of A0
  measures "d148" diameter of A1
  measures "d149" diameter of A2
extrude "Extrusion15" cut sketch "Sketch17" against normal blind 2
extrude "Extrusion16" add sketch "Sketch14" along normal blind 6
extrude "Extrusion17" add sketch "Sketch6" along normal blind 2 contours L96 L95 L94 L93 | L100 L99 L98 L97 | L104 L103 L102 L101
extrude "Extrusion18" add sketch "Sketch6" along normal blind 8 contours L100 L99 L98 L97 | L104 L103 L102 L101
extrude "Extrusion19" add sketch "Sketch6" along normal blind 10 contours A6 L89 | L89 A6 | A7
fillet "Fillet1" radius 0.5 2 edges at (-9, 6.4877, 11) (-17, -6, 11)
extrude "Extrusion20" add sketch "Sketch6" along normal up to next contours L141 L140 L139 L138 | L145 L144 L143 L142 | L149 L148 L147 L146 | L153 L152 L151 L150 | L157 L156 L155 L154 | L161 L160 L159 L158 | L165 L164 L163 L162 | L169 L168 L167 L166
extrude "Extrusion21" add sketch "Sketch6" along normal blind 3.5 contours L108 L107 L106 L105 | L113 L112 L111 L110 | L117 L116 L115 L114 | L121 L120 L119 L118 | L125 L124 L123 L122 | L129 L128 L127 L126 | L133 L132 L131 L130 | L137 L136 L135 L134
sketch "Sketch18" plane through (1.0618, 6.2177, 1) normal (1, 0, 0) x (0, 0, -1)
  line L0 (0, 0.5) -> (-3.5, 0.5) projected
  line L1 (0, 0) -> (-3.5, 0) projected
  line L2 (-3.5, 0.5) -> (-3, 0.5)
  line L3 (-3, 0.5) -> (-3, 0)
  line L4 (-3, 0) -> (-3.5, 0)
  line L5 (-3.5, 0) -> (-3.5, 0.5)
  line L6 (-3.5, -1.5) -> (-3, -1.5)
  line L7 (-3, -1.5) -> (-3, -2)
  line L8 (-3, -2) -> (-3.5, -2)
  line L9 (-3.5, -2) -> (-3.5, -1.5)
  line L10 (-3.5, -3.5) -> (-3, -3.5)
  line L11 (-3, -3.5) -> (-3, -4)
  line L12 (-3, -4) -> (-3.5, -4)
  line L13 (-3.5, -4) -> (-3.5, -3.5)
  line L14 (-3.5, -5.5) -> (-3, -5.5)
  line L15 (-3, -5.5) -> (-3, -6)
  line L16 (-3, -6) -> (-3.5, -6)
  line L17 (-3.5, -6) -> (-3.5, -5.5)
  line L18 (-3.5, -7.5) -> (-3, -7.5)
  line L19 (-3, -7.5) -> (-3, -8)
  line L20 (-3, -8) -> (-3.5, -8)
  line L21 (-3.5, -8) -> (-3.5, -7.5)
  line L22 (-3.5, -9.5) -> (-3, -9.5)
  line L23 (-3, -9.5) -> (-3, -10)
  line L24 (-3, -10) -> (-3.5, -10)
  line L25 (-3.5, -10) -> (-3.5, -9.5)
  line L26 (-3.5, -11.5) -> (-3, -11.5)
  line L27 (-3, -11.5) -> (-3, -12)
  line L28 (-3, -12) -> (-3.5, -12)
  line L29 (-3.5, -12) -> (-3.5, -11.5)
  line L30 (-3.5, -13.5) -> (-3, -13.5)
  line L31 (-3, -13.5) -> (-3, -14)
  line L32 (-3, -14) -> (-3.5, -14)
  line L33 (-3.5, -14) -> (-3.5, -13.5)
  point P0 (1, -6.2177)
  dimension "d209" = 2
  constraints: 64 end point, 2 parallel, 1 collinear, 1 horizontal, 1 perpendicular, 1 point on line, 1 vertical, 55 other
  measures "d209" distance of L3.end L7.end
extrude "Extrusion22" add sketch "Sketch18" along normal blind 7
sketch "Sketch19" plane through (0, 0, 4.5) normal (0, 0, 1) x (1, 0, 0)
  line L0 (8.0618, -7.2823) -> (7.5618, -7.2823)
  line L1 (7.5618, -7.2823) -> (7.5618, -7.7823)
  line L2 (7.5618, -7.7823) -> (8.0618, -7.7823)
  line L3 (8.0618, -7.7823) -> (8.0618, -7.2823)
  line L4 (8.0618, -5.2823) -> (7.5618, -5.2823)
  line L5 (7.5618, -5.2823) -> (7.5618, -5.7823)
  line L6 (7.5618, -5.7823) -> (8.0618, -5.7823)
  line L7 (8.0618, -5.7823) -> (8.0618, -5.2823)
  line L8 (8.0618, -3.2823) -> (7.5618, -3.2823)
  line L9 (7.5618, -3.2823) -> (7.5618, -3.7823)
  line L10 (7.5618, -3.7823) -> (8.0618, -3.7823)
  line L11 (8.0618, -3.7823) -> (8.0618, -3.2823)
  line L12 (8.0618, -1.2823) -> (7.5618, -1.2823)
  line L13 (7.5618, -1.2823) -> (7.5618, -1.7823)
  line L14 (7.5618, -1.7823) -> (8.0618, -1.7823)
  line L15 (8.0618, -1.7823) -> (8.0618, -1.2823)
  line L16 (8.0618, 0.7177) -> (7.5618, 0.7177)
  line L17 (7.5618, 0.7177) -> (7.5618, 0.2177)
  line L18 (7.5618, 0.2177) -> (8.0618, 0.2177)
  line L19 (8.0618, 0.2177) -> (8.0618, 0.7177)
  line L20 (8.0618, 2.7177) -> (7.5618, 2.7177)
  line L21 (7.5618, 2.7177) -> (7.5618, 2.2177)
  line L22 (7.5618, 2.2177) -> (8.0618, 2.2177)
  line L23 (8.0618, 2.2177) -> (8.0618, 2.7177)
  line L24 (8.0618, 4.7177) -> (7.5618, 4.7177)
  line L25 (7.5618, 4.7177) -> (7.5618, 4.2177)
  line L26 (7.5618, 4.2177) -> (8.0618, 4.2177)
  line L27 (8.0618, 4.2177) -> (8.0618, 4.7177)
  line L28 (8.0618, 6.7177) -> (7.5618, 6.7177)
  line L29 (7.5618, 6.7177) -> (7.5618, 6.2177)
  line L30 (7.5618, 6.2177) -> (8.0618, 6.2177)
  line L31 (8.0618, 6.2177) -> (8.0618, 6.7177)
  point P0 (0, 0)
  dimension "d216" = 0.5
  dimension "d217" = 0.5
  dimension "d220" = 2
  constraints: 64 end point, 2 parallel, 1 collinear, 1 horizontal, 1 perpendicular, 1 vertical, 55 other
  measures "d216" distance of L2.end L1.end
  measures "d217" distance of L1.end L0.end
  measures "d220" distance of L1.end L5.end
extrude "Extrusion23" add sketch "Sketch19" along normal up to next
sketch "Sketch20" plane through (0, 0, 0) normal (0, 0, -1) x (-1, 0, 0)
  line L0 (-21.65, -21.65) -> (-21.65, 21.65) projected
  line L1 (-21.65, 21.65) -> (21.4768, 21.65) construction
  line L2 (21.4768, 21.65) -> (21.4768, -21.65) construction
  line L3 (21.4768, -21.65) -> (-21.65, -21.65) construction
  line L4 (-21.65, -21.65) -> (-21.65, 21.65) construction
  point P0 (0, 0)
  constraints: 1 coincident, 2 other